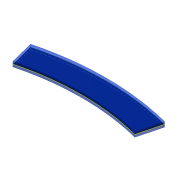
# Autodesk Inventor part: Midsurf
Saved by Autodesk Inventor 2014 (Build 180170000, 170)
## iProperties
Created: 2014-01-15
Part Number: Midsurf
Material: Generic
Document SubType Name: Modeling
Designer: Yogesh
Density: 1 g/cm^3
Appearance: Clear - Blue
Author: Yogesh
Autodesk Inventor part; units mm, degrees
ref_plane "YZ Plane" through (0, 0, 0) normal (1, 0, 0) x (0, 1, 0)
ref_plane "XZ Plane" through (0, 0, 0) normal (0, 1, 0) x (-1, 0, 0)
sketch "Sketch1" plane through (0, 0, 0) normal (0, 0, 1) x (1, 0, 0)
  arc A0 (50, 0) -> (0, 0) centre (25, -96.8246) ccw
  arc A1 (52.5042, 9.6987) -> (-2.5042, 9.6987) centre (25, -96.8246) ccw
  line L0 (-2.5042, 9.6987) -> (0, 0)
  line L1 (50, 0) -> (52.5042, 9.6987)
  constraints: 5 point on circle, 4 end point, 2 centre point
ref_plane "Work Plane1" through (0, 0, -100) normal (0, 0, 1) x (1, 0, 0)
extrude "Extrusion1" add sketch "Sketch1" against normal blind 2
surface_offset "OffsetSrf2"
body "Solid2"
body "Srf2"
